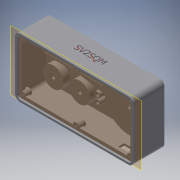
# Autodesk Inventor part: box
Saved by Autodesk Inventor 2017.3 (Build 213257000, 257)
## iProperties
Created: 2021-12-05
Part Number: box
Material: Generic
Document SubType Name: Modeling
Designer: TEOS
Density: 1 g/cm^3
Appearance: Default
Author: TEOS
Autodesk Inventor part; units mm, degrees
ref_plane "YZ Plane" through (0, 0, 0) normal (1, 0, 0) x (0, 1, 0)
ref_plane "XZ Plane" through (0, 0, 0) normal (0, 1, 0) x (-1, 0, 0)
ref_plane "XY Plane" through (0, 0, 0) normal (0, 0, 1) x (1, 0, 0)
sketch "Sketch1" plane through (0, 0, 0) normal (0, 1, 0) x (-1, 0, 0)
  line L0 (82, -45) -> (-82, -45)
  line L1 (-90, -37) -> (-90, 37)
  line L2 (-82, 45) -> (82, 45)
  line L3 (90, 37) -> (90, -37)
  arc A0 (82, -45) -> (90, -37) centre (82, -37) ccw
  arc A1 (90, 37) -> (82, 45) centre (82, 37) ccw
  arc A2 (-90, -37) -> (-82, -45) centre (-82, -37) ccw
  arc A3 (-82, 45) -> (-90, 37) centre (-82, 37) ccw
  line L4 (-82, -42) -> (82, -42)
  arc A4 (82, -42) -> (87, -37) centre (82, -37) ccw
  line L5 (87, -37) -> (87, 37)
  arc A5 (87, 37) -> (82, 42) centre (82, 37) ccw
  line L6 (82, 42) -> (-82, 42)
  arc A6 (-82, 42) -> (-87, 37) centre (-82, 37) ccw
  line L7 (-87, 37) -> (-87, -37)
  arc A7 (-87, -37) -> (-82, -42) centre (-82, -37) ccw
  point P0 (0, 0)
  point P1 (90, -45)
  point P2 (-90, -45)
  point P3 (90, 45)
  dimension "d0" = 180
  dimension "d1" = 90
  dimension "d2" = 8
  dimension "d3" = 3
  dimension "d24" = 90
  dimension "d25" = 45
  constraints: 16 end point, 16 point on circle, 8 centre point, 8 tangent, 6 point on line, 4 parallel, 3 equal radius, 2 perpendicular, 1 horizontal, 7 other
  measures "d0" distance of point (90, -45) point (-90, -45)
  measures "d1" distance of point (90, 45) point (90, -45)
  measures "d2" radius of A0
  measures "d3" distance between parallel lines of L0 L4
  measures "d24" distance from line of L1 point (0, 0)
  measures "d25" distance from line of point (0, 0) L0
extrude "Extrusion1" add sketch "Sketch1" along normal blind 45
sketch "Sketch2" plane through (0, 45, 0) normal (0, 1, 0) x (1, 0, 0)
  line L0 (82, 45) -> (-82, 45) projected
  arc A0 (-82, 45) -> (-90, 37) centre (-82, 37) ccw projected
  line L1 (-90, 37) -> (-90, -37) projected
  arc A1 (-90, -37) -> (-82, -45) centre (-82, -37) ccw projected
  line L2 (-82, -45) -> (82, -45) projected
  arc A2 (82, -45) -> (90, -37) centre (82, -37) ccw projected
  line L3 (90, -37) -> (90, 37) projected
  arc A3 (90, 37) -> (82, 45) centre (82, 37) ccw projected
  circle A4 centre (48.5, 3.5) radius 34
  circle A5 centre (-67, 22) radius 12.5
  circle A6 centre (-27, 22) radius 12.5
  line L4 (-90, 22) -> (90, 22) construction
  line L5 (20.5, -25.0657) -> (20.5, -34.5)
  line L6 (20.5, -34.5) -> (-79.5, -34.5)
  line L7 (-79.5, -34.5) -> (-79.5, -4.5)
  arc A7 (9.3082, -4.5) -> (20.5, -25.0657) centre (48.5, 3.5) ccw
  line L8 (-79.5, -4.5) -> (9.3082, -4.5)
  line L9 (-29.5, -4.5) -> (-29.5, -34.5)
  line L10 (-33.5, -4.5) -> (-33.5, -34.5)
  line L11 (-25.5, -4.5) -> (-25.5, -34.5)
  point P0 (0, 0)
  dimension "d6" = 68
  dimension "d7" = 41.5
  dimension "d8" = 41.5
  dimension "d9" = 25
  dimension "d10" = 25
  dimension "d11" = 23
  dimension "d12" = 23
  dimension "d13" = 40
  dimension "d14" = 100
  dimension "d15" = 30
  dimension "d16" = 10.5
  dimension "d17" = 10.5
  dimension "d18" = 80
  dimension "d19" = 50
  dimension "d20" = 8
  dimension "d21" = 4
  constraints: 16 end point, 9 point on line, 4 centre point, 4 perpendicular, 2 parallel, 2 point on circle, 1 coincident, 1 horizontal, 1 midpoint
  measures "d6" diameter of A4
  measures "d7" distance from line of L3 A4.centre
  measures "d8" distance from line of L0 A4.centre
  measures "d9" diameter of A6
  measures "d10" diameter of A5
  measures "d11" distance between parallel lines of L0 L4
  measures "d12" distance of A5.centre L4.start
  measures "d13" distance of A6.centre A5.centre
  measures "d14" distance of L5.end L6.end
  measures "d15" distance of L6.end L7.end
  measures "d16" distance between parallel lines of L7 L1
  measures "d17" distance between parallel lines of L2 L6
  measures "d18" diameter of A7
  measures "d19" distance between parallel lines of L7 L9
  measures "d20" distance between parallel lines of L11 L10
  measures "d21" distance between parallel lines of L10 L9
extrude "Extrusion2" add sketch "Sketch2" along normal blind 3 contours A3 L3 A2 L2 A1 L1 A0 L0 | L6 L9 L8 L11 | L6 L10 L8 L9
sketch "Sketch3" plane through (0, 45, 0) normal (0, -1, 0) x (1, 0, 0)
  circle A0 centre (-67, -22) radius 12.5 projected
  circle A1 centre (-27, -22) radius 12.5 projected
  line L0 (-25.5, 34.5) -> (20.5, 34.5) projected
  line L1 (20.5, 34.5) -> (20.5, 25.0657) projected
  arc A2 (20.5, 25.0657) -> (9.3082, 4.5) centre (48.5, -3.5) ccw projected
  line L2 (9.3082, 4.5) -> (-25.5, 4.5) projected
  line L3 (-25.5, 4.5) -> (-25.5, 34.5) projected
  line L4 (-33.5, 4.5) -> (-79.5, 4.5) projected
  line L5 (-79.5, 4.5) -> (-79.5, 34.5) projected
  line L6 (-79.5, 34.5) -> (-33.5, 34.5) projected
  line L7 (-33.5, 34.5) -> (-33.5, 4.5) projected
  circle A3 centre (48.5, -3.5) radius 34 projected
  arc A4 (82, -42) -> (87, -37) centre (82, -37) ccw projected
  line L8 (87, -37) -> (87, 37) projected
  arc A5 (87, 37) -> (82, 42) centre (82, 37) ccw projected
  line L9 (82, 42) -> (-82, 42) projected
  arc A6 (-82, 42) -> (-87, 37) centre (-82, 37) ccw projected
  line L10 (-87, 37) -> (-87, -37) projected
  arc A7 (-87, -37) -> (-82, -42) centre (-82, -37) ccw projected
  line L11 (-82, -42) -> (82, -42) projected
  circle A8 centre (48.5, -3.5) radius 37
  arc A9 (23.5, 23.7764) -> (11.5541, -5.5) centre (48.5, -3.5) ccw
  line L12 (23.5, 23.7764) -> (23.5, 37.5)
  line L13 (23.5, 37.5) -> (-28.5, 37.5)
  line L14 (-28.5, 1.5) -> (11.5541, -5.5)
  line L15 (-82.5, 1.5) -> (-30.5, 1.5)
  line L16 (-30.5, 37.5) -> (-82.5, 37.5)
  line L17 (-82.5, 37.5) -> (-82.5, 1.5)
  circle A10 centre (-27, -22) radius 15.5
  circle A11 centre (-67, -22) radius 15.5
  line L18 (-28.5, 1.5) -> (-30.5, 1.5)
  line L19 (-28.5, 37.5) -> (-30.5, 37.5)
  point P0 (0, 0)
  dimension "d26" = 3
  dimension "d27" = 3
  dimension "d28" = 3
  dimension "d29" = 3
  dimension "d30" = 3
  constraints: 16 end point, 4 centre point, 2 point on circle, 3 other
  measures "d26" radial gap between concentric circles of A3 A8
  measures "d27" radial gap between concentric circles of A2 A9
  measures "d28" distance between parallel lines of L4 L15
  measures "d29" radial gap between concentric circles of A1 A10
  measures "d30" radial gap between concentric circles of A0 A11
extrude "Extrusion3" add sketch "Sketch3" along normal blind 7 contours A8 | A8 L14 L18 L15 L17 L16 L19 L13 L12 | A10 | A11
sketch "Sketch4" plane through (0, 38, 0) normal (0, -1, 0) x (1, 0, 0)
  circle A0 centre (48.5, -3.5) radius 34 projected
  line L0 (-79.5, 4.5) -> (-79.5, 34.5) projected
  line L1 (-79.5, 34.5) -> (-33.5, 34.5) projected
  line L2 (-33.5, 34.5) -> (-33.5, 4.5) projected
  line L3 (-33.5, 4.5) -> (-79.5, 4.5) projected
  line L4 (20.5, 34.5) -> (20.5, 25.0657) projected
  arc A1 (20.5, 25.0657) -> (9.3082, 4.5) centre (48.5, -3.5) ccw projected
  line L5 (9.3082, 4.5) -> (-25.5, 4.5) projected
  line L6 (-25.5, 4.5) -> (-25.5, 34.5) projected
  line L7 (-25.5, 34.5) -> (20.5, 34.5) projected
  line L8 (23.5, 23.7764) -> (23.5, 37.5) projected
  line L9 (23.5, 37.5) -> (-82.5, 37.5) projected
  line L10 (-82.5, 37.5) -> (-82.5, 1.5) projected
  line L11 (-28.5, 1.5) -> (11.5541, -5.5) projected
  arc A2 (11.5541, -5.5) -> (23.5, 23.7764) centre (48.5, -3.5) ccw projected
  circle A3 centre (-27, -22) radius 12.5 projected
  circle A4 centre (-27, -22) radius 15.5 projected
  circle A5 centre (-67, -22) radius 12.5 projected
  circle A6 centre (-67, -22) radius 15.5 projected
  circle A7 centre (48.5, -3.5) radius 37
  line L12 (-82.5, 1.5) -> (-28.5, 1.5) projected
  point P0 (0, 0)
  constraints: 1 coincident, 3 other
extrude "Extrusion4" add sketch "Sketch4" along normal blind 3 contours A0 | A7 L11 L12 L10 L9 L8 | A2 A7 | A3 | A4 | A5 | A6
sketch "Sketch5" plane through (0, 35, 0) normal (0, -1, 0) x (1, 0, 0)
  circle A0 centre (-27, -22) radius 15.5 projected
  circle A1 centre (-67, -22) radius 15.5 projected
  line L0 (-79.5, 34.5) -> (-33.5, 34.5) projected
  line L1 (-33.5, 34.5) -> (-33.5, 4.5) projected
  line L2 (-33.5, 4.5) -> (-79.5, 4.5) projected
  line L3 (-79.5, 4.5) -> (-79.5, 34.5) projected
  arc A2 (20.5, 25.0657) -> (9.3082, 4.5) centre (48.5, -3.5) ccw projected
  line L4 (9.3082, 4.5) -> (-25.5, 4.5) projected
  line L5 (-25.5, 4.5) -> (-25.5, 34.5) projected
  line L6 (-25.5, 34.5) -> (20.5, 34.5) projected
  line L7 (20.5, 34.5) -> (20.5, 25.0657) projected
  line L8 (23.5, 23.7764) -> (23.5, 37.5) projected
  line L9 (23.5, 37.5) -> (-82.5, 37.5) projected
  line L10 (-82.5, 37.5) -> (-82.5, 1.5) projected
  line L11 (-28.5, 1.5) -> (11.5541, -5.5) projected
  arc A3 (11.5541, -5.5) -> (23.5, 23.7764) centre (48.5, -3.5) ccw projected
  line L12 (-82.5, 1.5) -> (-28.5, 1.5) projected
  point P0 (0, 0)
hole "Hole1" at (48.5, 35, -3.5) at (-27, 35, -22) at (-67, 35, -22) direction (0, 1, 0) diameter 6 end through all
chamfer "Chamfer1" distance 1 angle 45 8 edges at (87.6569, 48, 42.6569) (90, 48, 0) (87.6569, 48, -42.6569) (0, 48, -45) (-87.6569, 48, -42.6569) (-90, 48, 0) (-87.6569, 48, 42.6569) (0, 48, 45)
ref_plane "Work Plane1" through (0, 3, 0) normal (0, -1, 0) x (1, 0, 0)
sketch "Sketch7" plane through (0, 3, 0) normal (0, -1, 0) x (1, 0, 0)
  line L0 (82, -42) -> (-82, -42) projected
  arc A0 (-82, 42) -> (-87, 37) centre (-82, 37) ccw projected
  line L1 (-82, -32) -> (-82, 32)
  line L2 (82, 32) -> (82, -32)
  line L3 (82, 42) -> (-82, 42) projected
  arc A1 (77, 37) -> (82, 32) centre (82, 37) ccw
  arc A2 (82, -32) -> (77, -37) centre (82, -37) ccw
  arc A3 (-82, 32) -> (-77, 37) centre (-82, 37) ccw
  arc A4 (-82, 42) -> (-82.5, 41.9749) centre (-82, 37) ccw
  arc A5 (-86.9749, 37.5) -> (-87, 37) centre (-82, 37) ccw
  arc A6 (-77, -37) -> (-82, -32) centre (-82, -37) ccw
  arc A7 (-83.1803, -41.8587) -> (-82, -42) centre (-82, -37) ccw
  arc A8 (5, -37) -> (-5, -37) centre (0, -37) ccw
  arc A9 (-5, 37) -> (5, 37) centre (0, 37) ccw
  line L4 (77, -37) -> (5, -37)
  line L5 (-5, -37) -> (-77, -37)
  line L6 (-77, 37) -> (-5, 37)
  line L7 (5, 37) -> (77, 37)
  line L8 (87, 37) -> (87, -37) projected
  arc A10 (82, -42) -> (87, -37) centre (82, -37) ccw projected
  arc A11 (87, 37) -> (82, 42) centre (82, 37) ccw projected
  line L9 (-82, 42) -> (82, 42) projected
  arc A12 (-82, 42) -> (-87, 37) centre (-82, 37) ccw projected
  line L10 (-87, -37) -> (-87, 37) projected
  arc A13 (-87, -37) -> (-82, -42) centre (-82, -37) ccw projected
  circle A14 centre (82, -37) radius 5
  circle A15 centre (-82, -37) radius 5
  point P0 (0, 0)
  dimension "d65" = 5
  dimension "d66" = 5
  dimension "d67" = 5
  dimension "d68" = 5
  constraints: 19 point on circle, 15 end point, 9 centre point, 5 coincident, 5 parallel, 2 horizontal, 2 perpendicular, 2 vertical alignment, 6 other
  measures "d65" distance between parallel lines of L0 L5
  measures "d66" distance between parallel lines of L0 L4
  measures "d67" radius of A8
  measures "d68" distance from line of L0 A8.centre
extrude "Extrusion5" add sketch "Sketch7" against normal blind 10 contours A14 A2 A10 | L0 A15 L5 A8 L4 A14 | A7 A13 A15 A6 | A14 L2 A1 L7 A9 L6 A3 L1 A15 L10 A0 L3 A11 L8
sketch "Sketch8" plane through (0, 3, 0) normal (0, -1, 0) x (1, 0, 0)
  arc A0 (-77, -37) -> (-82, -32) centre (-82, -37) ccw projected
  line L0 (-82, -32) -> (-82, 32) projected
  arc A1 (-82, 32) -> (-77, 37) centre (-82, 37) ccw projected
  line L1 (-77, 37) -> (-5, 37) projected
  arc A2 (-5, 37) -> (5, 37) centre (0, 37) ccw projected
  line L2 (5, 37) -> (77, 37) projected
  arc A3 (77, 37) -> (82, 32) centre (82, 37) ccw projected
  line L3 (82, 32) -> (82, -32) projected
  arc A4 (82, -32) -> (77, -37) centre (82, -37) ccw projected
  line L4 (77, -37) -> (5, -37) projected
  arc A5 (5, -37) -> (-5, -37) centre (0, -37) ccw projected
  line L5 (-5, -37) -> (-77, -37) projected
  line L6 (82, -42) -> (-82, -42) projected
  arc A6 (82, -42) -> (87, -37) centre (82, -37) ccw projected
  line L7 (87, 37) -> (87, -37) projected
  arc A7 (87, 37) -> (82, 42) centre (82, 37) ccw projected
  line L8 (-82, 42) -> (82, 42) projected
  arc A8 (-82, 42) -> (-87, 37) centre (-82, 37) ccw projected
  line L9 (-87, -37) -> (-87, 37) projected
  arc A9 (-87, -37) -> (-82, -42) centre (-82, -37) ccw projected
  arc A10 (5, -37) -> (-5, -37) centre (0, -37) ccw projected
  point P0 (0, 0)
  constraints: 6 coincident
hole "Hole2" at (82, 3, 37) at (0, 3, 37) at (0, 3, -37) at (82, 3, -37) at (-82, 3, -37) at (-82, 3, 37) direction (0, 1, 0) diameter 2 depth 15 tip angle 118
chamfer "Chamfer2" distance 5 angle 45 6 edges at (-41, 13, 37) (41, 13, 37) (82, 13, 0) (41, 13, -37) (-41, 13, -37) (-82, 13, 0)
sketch "Sketch10" plane through (82, 0, -45) normal (0, 0, -1) x (-1, 0, 0)
  line L0 (18.0171, 20) -> (24.0171, 20) projected
  line L1 (24.0171, 20) -> (26.0171, 18) projected
  line L2 (26.0171, 18) -> (26.0171, 11) projected
  line L3 (26.0171, 11) -> (16.0171, 11) projected
  line L4 (16.0171, 11) -> (16.0171, 18) projected
  line L5 (16.0171, 18) -> (18.0171, 20) projected
  line L6 (15.0171, 10) -> (27.0171, 10) projected
  line L7 (27.0171, 10) -> (27.0171, 21) projected
  line L8 (15.0171, 21) -> (27.0171, 21) projected
  line L9 (15.0171, 10) -> (15.0171, 21) projected
  line L10 (27.0171, 9) -> (15.0171, 9)
  line L11 (14.0171, 10) -> (14.0171, 21)
  line L12 (15.0171, 22) -> (27.0171, 22)
  line L13 (28.0171, 21) -> (28.0171, 10)
  arc A0 (27.0171, 9) -> (28.0171, 10) centre (27.0171, 10) ccw
  arc A1 (28.0171, 21) -> (27.0171, 22) centre (27.0171, 21) ccw
  arc A2 (15.0171, 22) -> (14.0171, 21) centre (15.0171, 21) ccw
  arc A3 (14.0171, 10) -> (15.0171, 9) centre (15.0171, 10) ccw
  point P0 (82, 0)
  dimension "d69" = 1
  dimension "d70" = 1
  constraints: 8 end point, 8 point on circle, 8 tangent, 4 centre point, 3 equal radius, 3 other
  measures "d69" distance between parallel lines of L6 L10
  measures "d70" radius of A0
extrude "Extrusion6" cut sketch "Sketch10" against normal blind 10 contours L0 L1 L2 L3 L4 L5 | L9 L8 L7 L6 | L10 A3 L11 A2 L12 A1 L13 A0
sketch "Sketch11" plane through (-82, 0, 45) normal (0, 0, 1) x (1, 0, 0)
  line L0 (58.9181, 30.2232) -> (103.8593, 30.2232) construction
  line L1 (103.8593, 30.2232) -> (103.8593, 18.9844) construction
  line L2 (103.8593, 18.9844) -> (58.9181, 18.9844) construction
  line L3 (58.9181, 18.9844) -> (58.9181, 30.2232) construction
  line L4 (164, 48) -> (0, 48) projected
  line L5 (169, 3) -> (164, 3) projected
  line L6 (0, 48) -> (164, 3)
  line L7 (164, 3) -> (164, 48)
  line L8 (0, 47) -> (164, 47) projected
  line L9 (164, 48) -> (0, 3)
  spline S0 degree 2 poles (62.2436, 21.1329) (61.2935, 21.1329) (59.9604, 21.5299) (59.3719, 21.8136) knots 0 0 0 1 2 2 2
  line L10 (59.3719, 21.8136) -> (59.3719, 23.2743)
  line L11 (59.3719, 23.2743) -> (59.457, 23.2743)
  spline S1 degree 2 poles (59.457, 23.2743) (60.0313, 22.7354) (61.4849, 22.1398) (62.1585, 22.1398) knots 0 0 0 1 2 2 2
  spline S2 degree 2 poles (62.1585, 22.1398) (63.1229, 22.1398) (64.1085, 22.941) (64.1085, 23.6005) knots 0 0 0 1 2 2 2
  spline S3 degree 2 poles (64.1085, 23.6005) (64.1085, 24.1252) (63.5909, 24.7775) (63.0307, 24.9406) knots 0 0 0 1 2 2 2
  spline S4 degree 2 poles (63.0307, 24.9406) (62.6265, 25.0541) (61.9529, 25.2101) (61.4495, 25.3377) knots 0 0 0 1 2 2 2
  spline S5 degree 2 poles (61.4495, 25.3377) (60.9957, 25.4582) (60.2795, 25.8199) (60.003, 26.1106) knots 0 0 0 1 2 2 2
  spline S6 degree 2 poles (60.003, 26.1106) (59.7335, 26.4013) (59.4357, 27.1813) (59.4357, 27.6918) knots 0 0 0 1 2 2 2
  spline S7 degree 2 poles (59.4357, 27.6918) (59.4357, 28.7554) (61.0949, 30.1949) (62.3784, 30.1949) knots 0 0 0 1 2 2 2
  spline S8 degree 2 poles (62.3784, 30.1949) (63.1158, 30.1949) (64.4205, 29.9041) (64.9807, 29.6276) knots 0 0 0 1 2 2 2
  line L12 (64.9807, 29.6276) -> (64.9807, 28.2378)
  line L13 (64.9807, 28.2378) -> (64.8956, 28.2378)
  spline S9 degree 2 poles (64.8956, 28.2378) (64.4772, 28.6207) (63.1725, 29.188) (62.4564, 29.188) knots 0 0 0 1 2 2 2
  spline S10 degree 2 poles (62.4564, 29.188) (61.648, 29.188) (60.6482, 28.4293) (60.6482, 27.8124) knots 0 0 0 1 2 2 2
  spline S11 degree 2 poles (60.6482, 27.8124) (60.6482, 27.2593) (61.2367, 26.5998) (61.7898, 26.4509) knots 0 0 0 1 2 2 2
  spline S12 degree 2 poles (61.7898, 26.4509) (62.1585, 26.3517) (63.2293, 26.0964) (63.5838, 25.99) knots 0 0 0 1 2 2 2
  spline S13 degree 2 poles (63.5838, 25.99) (64.4843, 25.7135) (65.321, 24.6002) (65.321, 23.7848) knots 0 0 0 1 2 2 2
  spline S14 degree 2 poles (65.321, 23.7848) (65.321, 23.2672) (64.9027, 22.2745) (64.5269, 21.927) knots 0 0 0 1 2 2 2
  spline S15 degree 2 poles (64.5269, 21.927) (64.1085, 21.5441) (63.0449, 21.1329) (62.2436, 21.1329) knots 0 0 0 1 2 2 2
  line L14 (72.8514, 30.0389) -> (69.8378, 21.2889)
  line L15 (69.8378, 21.2889) -> (68.5828, 21.2889)
  line L16 (68.5828, 21.2889) -> (65.5692, 30.0389)
  line L17 (65.5692, 30.0389) -> (66.8172, 30.0389)
  line L18 (66.8172, 30.0389) -> (69.2422, 22.7708)
  line L19 (69.2422, 22.7708) -> (71.6673, 30.0389)
  line L20 (71.6673, 30.0389) -> (72.8514, 30.0389)
  line L21 (78.836, 21.2889) -> (73.44, 21.2889)
  line L22 (73.44, 21.2889) -> (73.44, 22.5297)
  spline S16 degree 2 poles (73.44, 22.5297) (74.0214, 23.0757) (75.0566, 24.0897) (75.553, 24.6357) knots 0 0 0 1 2 2 2
  spline S17 degree 2 poles (75.553, 24.6357) (76.5528, 25.7348) (77.2831, 27.0537) (77.2831, 27.7556) knots 0 0 0 1 2 2 2
  spline S18 degree 2 poles (77.2831, 27.7556) (77.2831, 28.1244) (77.0562, 28.6774) (76.8506, 28.8547) knots 0 0 0 1 2 2 2
  spline S19 degree 2 poles (76.8506, 28.8547) (76.645, 29.032) (76.1061, 29.2092) (75.7799, 29.2092) knots 0 0 0 1 2 2 2
  spline S20 degree 2 poles (75.7799, 29.2092) (75.4679, 29.2092) (74.8297, 29.0532) (74.539, 28.9327) knots 0 0 0 1 2 2 2
  spline S21 degree 2 poles (74.539, 28.9327) (74.2908, 28.8334) (73.8299, 28.5498) (73.6881, 28.4505) knots 0 0 0 1 2 2 2
  line L23 (73.6881, 28.4505) -> (73.6243, 28.4505)
  line L24 (73.6243, 28.4505) -> (73.6243, 29.6985)
  spline S22 degree 2 poles (73.6243, 29.6985) (73.9859, 29.8758) (75.2835, 30.2232) (75.865, 30.2232) knots 0 0 0 1 2 2 2
  spline S23 degree 2 poles (75.865, 30.2232) (77.0917, 30.2232) (78.4744, 28.9256) (78.4744, 27.8195) knots 0 0 0 1 2 2 2
  spline S24 degree 2 poles (78.4744, 27.8195) (78.4744, 27.3018) (78.2333, 26.4368) (78.0206, 26.068) knots 0 0 0 1 2 2 2
  spline S25 degree 2 poles (78.0206, 26.068) (77.8079, 25.6851) (77.191, 24.9335) (76.8506, 24.5719) knots 0 0 0 1 2 2 2
  spline S26 degree 2 poles (76.8506, 24.5719) (76.2975, 23.9692) (74.9432, 22.6787) (74.539, 22.3028) knots 0 0 0 1 2 2 2
  line L25 (74.539, 22.3028) -> (78.836, 22.3028)
  line L26 (78.836, 22.3028) -> (78.836, 21.2889)
  spline S27 degree 2 poles (82.6934, 21.1329) (81.7432, 21.1329) (80.4102, 21.5299) (79.8216, 21.8136) knots 0 0 0 1 2 2 2
  line L27 (79.8216, 21.8136) -> (79.8216, 23.2743)
  line L28 (79.8216, 23.2743) -> (79.9067, 23.2743)
  spline S28 degree 2 poles (79.9067, 23.2743) (80.4811, 22.7354) (81.9347, 22.1398) (82.6083, 22.1398) knots 0 0 0 1 2 2 2
  spline S29 degree 2 poles (82.6083, 22.1398) (83.5726, 22.1398) (84.5583, 22.941) (84.5583, 23.6005) knots 0 0 0 1 2 2 2
  spline S30 degree 2 poles (84.5583, 23.6005) (84.5583, 24.1252) (84.0406, 24.7775) (83.4805, 24.9406) knots 0 0 0 1 2 2 2
  spline S31 degree 2 poles (83.4805, 24.9406) (83.0763, 25.0541) (82.4027, 25.2101) (81.8992, 25.3377) knots 0 0 0 1 2 2 2
  spline S32 degree 2 poles (81.8992, 25.3377) (81.4454, 25.4582) (80.7293, 25.8199) (80.4527, 26.1106) knots 0 0 0 1 2 2 2
  spline S33 degree 2 poles (80.4527, 26.1106) (80.1833, 26.4013) (79.8855, 27.1813) (79.8855, 27.6918) knots 0 0 0 1 2 2 2
  spline S34 degree 2 poles (79.8855, 27.6918) (79.8855, 28.7554) (81.5447, 30.1949) (82.8281, 30.1949) knots 0 0 0 1 2 2 2
  spline S35 degree 2 poles (82.8281, 30.1949) (83.5656, 30.1949) (84.8703, 29.9041) (85.4304, 29.6276) knots 0 0 0 1 2 2 2
  line L29 (85.4304, 29.6276) -> (85.4304, 28.2378)
  line L30 (85.4304, 28.2378) -> (85.3453, 28.2378)
  spline S36 degree 2 poles (85.3453, 28.2378) (84.927, 28.6207) (83.6223, 29.188) (82.9061, 29.188) knots 0 0 0 1 2 2 2
  spline S37 degree 2 poles (82.9061, 29.188) (82.0978, 29.188) (81.098, 28.4293) (81.098, 27.8124) knots 0 0 0 1 2 2 2
  spline S38 degree 2 poles (81.098, 27.8124) (81.098, 27.2593) (81.6865, 26.5998) (82.2396, 26.4509) knots 0 0 0 1 2 2 2
  spline S39 degree 2 poles (82.2396, 26.4509) (82.6083, 26.3517) (83.679, 26.0964) (84.0335, 25.99) knots 0 0 0 1 2 2 2
  spline S40 degree 2 poles (84.0335, 25.99) (84.9341, 25.7135) (85.7708, 24.6002) (85.7708, 23.7848) knots 0 0 0 1 2 2 2
  spline S41 degree 2 poles (85.7708, 23.7848) (85.7708, 23.2672) (85.3524, 22.2745) (84.9766, 21.927) knots 0 0 0 1 2 2 2
  spline S42 degree 2 poles (84.9766, 21.927) (84.5583, 21.5441) (83.4947, 21.1329) (82.6934, 21.1329) knots 0 0 0 1 2 2 2
  spline S43 degree 2 poles (94.223, 19.1475) (93.9039, 19.0695) (93.209, 18.9844) (92.8615, 18.9844) knots 0 0 0 1 2 2 2
  spline S44 degree 2 poles (92.8615, 18.9844) (91.8759, 18.9844) (90.6492, 20.0834) (90.5925, 21.1045) knots 0 0 0 1 2 2 2
  spline S45 degree 2 poles (90.5925, 21.1045) (90.5145, 21.1045) (90.3798, 21.1045) (90.3231, 21.1045) knots 0 0 0 1 2 2 2
  spline S46 degree 2 poles (90.3231, 21.1045) (89.4367, 21.1045) (88.0115, 21.7072) (87.5009, 22.2958) knots 0 0 0 1 2 2 2
  spline S47 degree 2 poles (87.5009, 22.2958) (86.9975, 22.8772) (86.4586, 24.579) (86.4586, 25.6568) knots 0 0 0 1 2 2 2
  spline S48 degree 2 poles (86.4586, 25.6568) (86.4586, 26.7629) (87.0046, 28.4364) (87.508, 29.032) knots 0 0 0 1 2 2 2
  spline S49 degree 2 poles (87.508, 29.032) (88.0186, 29.6205) (89.4438, 30.2232) (90.3231, 30.2232) knots 0 0 0 1 2 2 2
  spline S50 degree 2 poles (90.3231, 30.2232) (91.2165, 30.2232) (92.6488, 29.5992) (93.1452, 29.032) knots 0 0 0 1 2 2 2
  spline S51 degree 2 poles (93.1452, 29.032) (93.6415, 28.4576) (94.1946, 26.7487) (94.1946, 25.6568) knots 0 0 0 1 2 2 2
  spline S52 degree 2 poles (94.1946, 25.6568) (94.1946, 23.955) (92.8686, 21.7427) (91.7128, 21.3527) knots 0 0 0 1 2 2 2
  spline S53 degree 2 poles (91.7128, 21.3527) (91.7412, 21.0265) (91.9114, 20.5018) (92.0461, 20.3529) knots 0 0 0 1 2 2 2
  spline S54 degree 2 poles (92.0461, 20.3529) (92.2092, 20.1685) (92.6559, 19.9983) (93.053, 19.9983) knots 0 0 0 1 2 2 2
  spline S55 degree 2 poles (93.053, 19.9983) (93.287, 19.9983) (93.9252, 20.1472) (94.067, 20.204) knots 0 0 0 1 2 2 2
  line L31 (94.067, 20.204) -> (94.223, 20.204)
  line L32 (94.223, 20.204) -> (94.223, 19.1475)
  spline S56 degree 2 poles (92.9821, 25.6568) (92.9821, 26.5289) (92.6063, 27.8691) (92.2659, 28.3087) knots 0 0 0 1 2 2 2
  spline S57 degree 2 poles (92.2659, 28.3087) (91.9185, 28.7625) (90.94, 29.2163) (90.3301, 29.2163) knots 0 0 0 1 2 2 2
  spline S58 degree 2 poles (90.3301, 29.2163) (89.6991, 29.2163) (88.7489, 28.7767) (88.3873, 28.3087) knots 0 0 0 1 2 2 2
  spline S59 degree 2 poles (88.3873, 28.3087) (88.0398, 27.862) (87.6711, 26.5077) (87.6711, 25.6568) knots 0 0 0 1 2 2 2
  spline S60 degree 2 poles (87.6711, 25.6568) (87.6711, 23.9337) (89.1176, 22.0972) (90.3301, 22.0972) knots 0 0 0 1 2 2 2
  spline S61 degree 2 poles (90.3301, 22.0972) (91.5427, 22.0972) (92.9821, 23.9337) (92.9821, 25.6568) knots 0 0 0 1 2 2 2
  line L33 (102.973, 21.2889) -> (101.8101, 21.2889)
  line L34 (101.8101, 21.2889) -> (101.8101, 28.8263)
  line L35 (101.8101, 28.8263) -> (99.5269, 23.6997)
  line L36 (99.5269, 23.6997) -> (98.8178, 23.6997)
  line L37 (98.8178, 23.6997) -> (96.5558, 28.8263)
  line L38 (96.5558, 28.8263) -> (96.5558, 21.2889)
  line L39 (96.5558, 21.2889) -> (95.4709, 21.2889)
  line L40 (95.4709, 21.2889) -> (95.4709, 30.0389)
  line L41 (95.4709, 30.0389) -> (97.0593, 30.0389)
  line L42 (97.0593, 30.0389) -> (99.2432, 25.1675)
  line L43 (99.2432, 25.1675) -> (101.3563, 30.0389)
  line L44 (101.3563, 30.0389) -> (102.973, 30.0389)
  line L45 (102.973, 30.0389) -> (102.973, 21.2889)
  point P0 (82, 0)
  constraints: 6 end point, 1 perpendicular, 2 other
emboss "Emboss1" sketch "Sketch11" operation cut depth 1.5 direction (0, 0, -1) contours L42 L43 L44 L45 L33 L34 L35 L36 L37 L38 L6 L40 L9 | L9 L40 L41 L42 | L16 L17 L18 L6 | L6 L18 L19 L14 L9 L16 | L38 L39 L40 L6 | L9 L14 L15 L16 | S51 S52 L6 S61 S56 S57 L9 | L9 S57 S58 S59 S48 S49 S50 S51 | L19 L20 L14 L6 | S52 S53 S54 S55 L31 L32 S43 S44 S45 S46 S47 L6 S60 S61 | S16 S17 L6 S24 S25 S26 L9 | L9 S26 L25 L26 L21 L22 S16 | S59 S60 L6 S47 S48 L9 | S17 S18 S19 S20 S21 L23 L24 S22 S23 S24 L6 | S32 L6 L9 | L9 L6 S40 S41 S42 S27 L27 L28 S28 S29 S30 S31 S32 | S39 S40 L6 L9 | L9 L6 S32 S33 S34 S35 L29 L30 S36 S37 S38 S39 | S0 L10 L11 S1 S2 S3 S4 S5 S6 S7 S8 L12 L13 S9 S10 S11 S12 S13 S14 S15
sketch "Sketch12" plane through (0, 45, 0) normal (0, -1, 0) x (1, 0, 0)
  circle A0 centre (-67, -22) radius 3 construction
  circle A1 centre (0, -12) radius 4.5
  circle A2 centre (0, -27) radius 4.5
  circle A3 centre (0, -12) radius 2.45
  circle A4 centre (0, -27) radius 2.45
  arc A5 (5, -37) -> (-5, -37) centre (0, -37) ccw projected
  line L0 (0, -37) -> (0, -6.1693)
  point P0 (0, 0)
  dimension "d75" = 9
  dimension "d76" = 9
  dimension "d77" = 4.9
  dimension "d78" = 4.9
  dimension "d79" = 15
  dimension "d81" = 10
  constraints: 4 centre point, 2 coincident, 2 end point, 2 point on line, 1 vertical
  measures "d75" diameter of A1
  measures "d76" diameter of A2
  measures "d77" diameter of A3
  measures "d78" diameter of A4
  measures "d79" distance of A2.centre A1.centre
  measures "d81" distance of L0.start A2.centre
extrude "Extrusion7" add sketch "Sketch12" along normal blind 10 contours A1 L0 A3 | L0 A3 A1 | A2 L0 A4 | L0 A4 A2
body "Solid1"
